line 10 cm 2mm cutter_v4 (Autodesk Fusion 360 design; units mm, degrees)
Autodesk Fusion 360 part; units mm, degrees
sketch "Sketch1" plane through (0, 0, 0) normal (0, 0, 1) x (1, 0, 0)
  line L0 (0, 114) -> (2, 114)
  line L1 (2, 0) -> (0, 0)
  line L2 (30.5953, -12.9847) -> (-37.9542, -12.9847)
  line L3 (-37.9542, -12.9847) -> (-37.9542, 117.0153)
  line L4 (-37.9542, 117.0153) -> (30.5953, 117.0153)
  line L5 (30.5953, 117.0153) -> (30.5953, -12.9847)
  line L6 (0, 0) -> (2, 0)
  line L7 (2, 0) -> (2, 100)
  line L8 (2, 100) -> (0, 100)
  line L9 (0, 100) -> (0, 0)
  circle A0 centre (-25.0399, 47.6257) radius 8.2184
  dimension "d2" = 2
  dimension "d5" = 68.5495
  dimension "d8" = 2
  dimension "d9" = 100
  dimension "d10" = 130
  dimension "d19" = 16.4367
  constraint coincident L1.end L6.start
  constraint horizontal L0
  constraint horizontal L1
  constraint horizontal L2
  constraint vertical L3
  constraint horizontal L4
  constraint vertical L5
  constraint horizontal L6
  constraint vertical L7
  constraint horizontal L8
  constraint vertical L9
  measures "d2" distance of L1.end L1.start
  measures "d5" distance of L2.start L2.end
  measures "d8" distance of L1.end L1.start
  measures "d9" distance of L1.end L8.end
  measures "d10" distance of L2.end L3.end
  measures "d19" diameter of A0
extrude "Extrude7" add sketch "Sketch1" along normal blind 3.176
